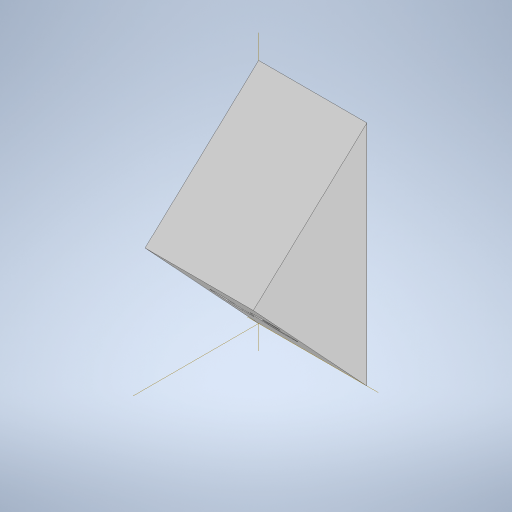
# Autodesk Inventor part: Triangle_V3
Saved by Autodesk Inventor 2023 (Build 270158000, 158)
## iProperties
Created: 2022-09-01
Part Number: Triangle_V3
Material: Generic
Document SubType Name: Modeling
Designer: brian
Density: 1 g/cm^3
Appearance: Default
Author: brian
Autodesk Inventor part; units mm, degrees
ref_plane "YZ Plane" through (0, 0, 0) normal (1, 0, 0) x (0, 1, 0)
ref_plane "XZ Plane" through (0, 0, 0) normal (0, 1, 0) x (-1, 0, 0)
ref_plane "XY Plane" through (0, 0, 0) normal (0, 0, 1) x (1, 0, 0)
sketch "Sketch1" plane through (0, 0, 0) normal (0, 0, 1) x (1, 0, 0)
  line L0 (0, 0) -> (185, 0)
  line L1 (185, 0) -> (185, 450)
  line L2 (185, 450) -> (0, 450)
  line L3 (0, 450) -> (0, 0)
  dimension "d0" = 185
  dimension "d1" = 450
  constraints: 8 end point, 2 parallel, 1 horizontal, 1 perpendicular
  measures "d0" distance of L0.start L0.end
  measures "d1" distance of L2.end L0.start
extrude "Extrusion1" add sketch "Sketch1" along normal blind 400
sketch "Sketch2" plane through (0, 0, 0) normal (-1, 0, 0) x (0, 0, 1)
  line L0 (0, 0) -> (0, 450) projected
  line L1 (0, 0) -> (194.069, 208.7157)
  line L2 (194.069, 208.7157) -> (0, 389.1658)
  line L3 (0, 0) -> (0, 389.1658)
  line L4 (0, 450) -> (0, 0) projected
  line L5 (0, 0) -> (400, 0) projected
  line L6 (400, 450) -> (400, 0) projected
  line L7 (0, 450) -> (400, 450) projected
  dimension "d4" = 265
  dimension "d5" = 90
  dimension "d6" = 285
  constraints: 6 end point, 1 collinear, 1 perpendicular, 1 point on line
  measures "d4" distance of L1.end L2.end
  measures "d5" angle of L2 L1
  measures "d6" distance of L0.start L1.end
extrude "Extrusion2" cut sketch "Sketch2" against normal blind 400 contours L1 L2 L0 L7 L6 L5
sketch "Sketch3" plane through (0, 208.7157, 194.069) normal (0, -0.6809437, 0.7323357) x (1, 0, 0)
  line L0 (34.9517, -115.3139) -> (34.9517, -157.3139)
  line L1 (48.9517, -171.3139) -> (58.9517, -171.3139)
  line L2 (48.9517, -101.3139) -> (54.9517, -101.3139)
  circle A0 centre (54.9517, -116.5313) radius 15.2174
  circle A1 centre (58.9517, -151.5313) radius 19.7826
  line L3 (58.9517, -131.7487) -> (54.9517, -131.7487)
  arc A2 (48.9517, -101.3139) -> (34.9517, -115.3139) centre (48.9517, -115.3139) ccw
  arc A3 (34.9517, -157.3139) -> (48.9517, -171.3139) centre (48.9517, -157.3139) ccw
  circle A4 centre (128.9517, -136.3139) radius 35
  circle A5 centre (128.9517, -136.3139) radius 17.5
  circle A6 centre (142.9517, -114.1089) radius 8.75
  circle A7 centre (142.9517, -158.5189) radius 8.75
  point P0 (0, -285)
  point P1 (0, 0)
  point P2 (34.9517, -101.3139)
  point P3 (34.9517, -171.3139)
  point P4 (34.9517, -136.3139)
  point P5 (135.9261, 202.4385)
  point P6 (135.9261, 232.0451)
  point P7 (145.2595, 246.8485)
  point P8 (145.2595, 187.6351)
  point P9 (52.5928, 252.2418)
  point P10 (56.5928, 182.2418)
  point P11 (138.285, -151.1172)
  point P12 (138.285, -121.5105)
  point P13 (147.6184, -106.7072)
  point P14 (147.6184, -165.9206)
  point P15 (58.9517, -171.3139)
  dimension "d12" = 30.4348
  dimension "d13" = 39.5652
  dimension "d9" = 70
  dimension "d10" = 24
  dimension "d11" = 20
  dimension "d14" = 15.2174
  dimension "d15" = 19.7826
  dimension "d16" = 14
  dimension "d17" = 70
  dimension "d18" = 35
  dimension "d19" = 17.5
  dimension "d20" = 17.5
  dimension "d21" = 14
  dimension "d22" = 70
  constraints: 8 end point, 6 centre point, 6 tangent, 4 point on circle, 4 point on line, 3 horizontal, 3 vertical alignment, 1 coincident, 1 equal radius, 1 horizontal alignment, 1 midpoint, 1 perpendicular, 1 vertical, 6 other
  measures "d9" distance of point (34.952, -101.314) point (34.952, -171.314)
  measures "d10" distance of point (34.952, -171.314) L1.end
  measures "d11" distance of point (34.952, -101.314) L2.end
  measures "d14" distance of L2.end point (54.952, -116.531)
  measures "d15" distance of L1.end point (58.952, -151.531)
  measures "d16" radius of A2
  measures "d17" diameter of A4
  measures "d18" diameter of A5
  measures "d19" diameter of A6
  measures "d20" diameter of A7
  measures "d21" horizontal distance of A4.centre A7.centre
  measures "d22" horizontal distance of point (58.952, -151.531) A4.centre
extrude "Extrusion3" cut sketch "Sketch3" against normal blind 10 contours A2 L2 A0 L3 A1 L1 A3 L0 | A0 | A1 | A6 A5 A7 A4 | A6 | A7 picked at (128.1694, -161.6024)
equation "\"d12\" = 0.434783 * d9"
equation "\"d13\" = d9 - d12"
equation "\"d10\" = 1.2 * d11"
equation "\"d11\" = 0.285714 * d9"
equation "\"d14\" = 0.5 * d12"
equation "\"d15\" = 0.5 * d13"
equation "\"d16\" = 0.2 * d9"
equation "\"d17\" = d9"
equation "\"d18\" = 0.5 * d17"
equation "\"d19\" = -0.5 * d18 + 0.5 * d17"
equation "\"d20\" = d19"
equation "\"d21\" = 0.2 * d17"
equation "\"d22\" = d9"
body "Solid1"
